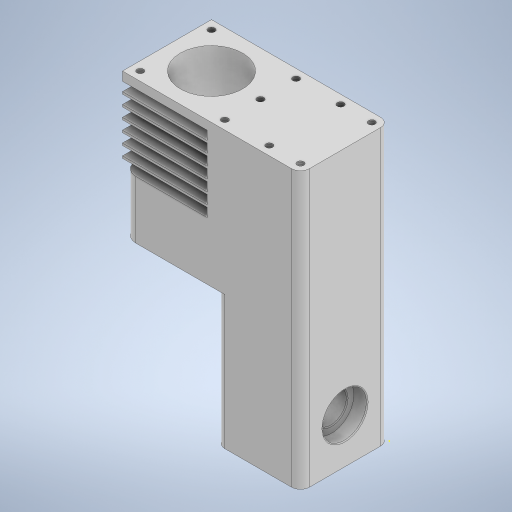
# Autodesk Inventor part: Hộp Piston
Saved by Autodesk Inventor 2023 (Build 270158000, 158)
## iProperties
Created: 2023-10-06
Part Number: Hộp Piston
Material: Generic
Document SubType Name: Modeling
Designer: huy20
Density: 1 g/cm^3
Appearance: Default
Author: huy20
Autodesk Inventor part; units mm, degrees
ref_plane "YZ Plane" through (0, 0, 0) normal (1, 0, 0) x (0, 1, 0)
ref_plane "XZ Plane" through (0, 0, 0) normal (0, 1, 0) x (-1, 0, 0)
sketch "Sketch1" plane through (0, 0, 0) normal (0, 0, 1) x (1, 0, 0)
  line L0 (0, 0) -> (19, 0)
  line L1 (0, 30) -> (0, 0)
  line L2 (0, 30) -> (-21, 30)
  line L3 (-21, 30) -> (-21, 62)
  line L4 (-21, 62) -> (19, 62)
  line L5 (19, 62) -> (19, 0)
  dimension "d0" = 32
  dimension "d1" = 21
  dimension "d2" = 30
  dimension "d3" = 40
  constraints: 12 end point, 2 horizontal, 2 perpendicular, 1 parallel
  measures "d0" distance of L2.end L3.end
  measures "d1" distance between parallel lines of L3 L1
  measures "d2" distance of L1.start L0.start
  measures "d3" distance of L3.end L4.end
extrude "Extrusion1" add sketch "Sketch1" along normal blind 20
sketch "Sketch2" plane through (-21, 30, 0) normal (0, -1, 0) x (1, 0, 0)
  circle A0 centre (10, 10) radius 7
  line L0 (0, 0) -> (21, 0) projected
  line L1 (0, 0) -> (0, 20) projected
  dimension "d6" = 14
  dimension "d7" = 10
  dimension "d8" = 10
  constraints: 1 centre point
  measures "d6" diameter of A0
  measures "d7" distance from line of L0 A0.centre
  measures "d8" distance from line of L1 A0.centre
extrude "Extrusion2" cut sketch "Sketch2" against normal through all
ref_plane "Work Plane1" through (-21, 60, 0) normal (0, 1, 0) x (1, 0, 0)
sketch "Sketch3" plane through (-21, 60, 0) normal (0, 1, 0) x (1, 0, 0)
  line L0 (0, 0) -> (0, -20) projected
  line L1 (21, 0) -> (0, 0)
  line L2 (0, 0) -> (0, -20)
  line L3 (0, -20) -> (19, -20)
  line L4 (2, -2) -> (20.5, -2)
  line L5 (18.5, -18) -> (2, -18)
  line L6 (2, -18) -> (2, -2)
  line L7 (20.5, -2) -> (21, -2)
  line L8 (18.5, -18) -> (19, -18)
  line L9 (19, -20) -> (19, -18)
  line L10 (21, -2) -> (21, 0)
  dimension "d12" = 2
  dimension "d13" = 2
  constraints: 20 end point, 6 perpendicular, 4 parallel, 1 horizontal, 1 other
  measures "d12" distance between parallel lines of L1 L4
  measures "d13" distance between parallel lines of L3 L5
extrude "Extrusion3" cut sketch "Sketch3" against normal blind 2
pattern_linear "Rectangular Pattern1" count 7 spacing 2.5 along (0, -1, 0) of "Extrusion3"
fillet "Fillet1" radius 3 16 edges at (-19, 59, 2) (-19, 56.5, 2) (-19, 54, 2) (-19, 51.5, 2) (-19, 49, 2) (-19, 46.5, 2) (-19, 44, 2) (-21, 36.5, 0) (-21, 36.5, 20) (-19, 44, 18) (-19, 46.5, 18) (-19, 49, 18) (-19, 51.5, 18) (-19, 54, 18) (-19, 56.5, 18) (-19, 59, 18)
fillet "Fillet2" radius 2 4 edges at (19, 31, 0) (19, 31, 20) (0, 15, 20) (0, 15, 0)
sketch "Sketch4" plane through (19, 0, 18) normal (1, 0, 0) x (0, 0, -1)
  line L0 (0, 0) -> (0, 62) construction
  line L1 (16, 0) -> (0, 0) construction
  line L2 (16, 62) -> (16, 0) construction
  line L3 (16, 62) -> (0, 62) construction
  circle A0 centre (8, 10) radius 3.5
  point P0 (18, 0)
  point P1 (8, 0)
  dimension "d21" = 7
  dimension "d22" = 10
  constraints: 1 centre point, 1 midpoint
  measures "d21" diameter of A0
  measures "d22" distance of point (8, 0) A0.centre
extrude "Extrusion4" cut sketch "Sketch4" against normal through all
sketch "Sketch5" plane through (-21, 62, 20) normal (0, 1, 0) x (1, 0, 0)
  circle A0 centre (10, 10) radius 7 projected
  arc A1 (38, 0) -> (40, 2) centre (38, 2) ccw projected
  line L0 (40, 18) -> (40, 2) projected
  arc A2 (40, 18) -> (38, 20) centre (38, 18) ccw projected
  line L1 (38, 20) -> (0, 20) projected
  line L2 (0, 20) -> (0, 0) projected
  line L3 (38, 0) -> (0, 0) projected
  line L4 (21, 18) -> (21, 2) projected
  point P0 (31, 18)
  point P1 (31, 2)
  point P2 (21, 10)
  point P3 (2, 18)
  point P4 (2, 2)
  dimension "d79" = 10
  dimension "d80" = 7
  dimension "d81" = 10
  dimension "d82" = 7
  dimension "d83" = 19
  dimension "d84" = 19
  dimension "d85" = 16
  dimension "d86" = 19
  dimension "d87" = 10
  dimension "d88" = 38
  constraints: 2 coincident
  measures "d79" distance of point (31, 18) L4.start
  measures "d80" distance of A2.centre point (31, 18)
  measures "d81" distance of point (31, 2) L4.end
  measures "d82" distance of A1.centre point (31, 2)
  measures "d83" distance of L4.end point (2, 2)
  measures "d84" distance of L4.start point (2, 18)
  measures "d85" distance of point (2, 2) point (2, 18)
  measures "d86" distance from line of point (21, 10) L0
  measures "d87" distance from line of point (21, 10) L1
  measures "d88" distance from line of point (2, 18) L0
hole "Hole1" at (0, 62, 2) at (-19, 62, 2) at (-19, 62, 18) at (0, 62, 18) at (10, 62, 18) at (17, 62, 18) at (17, 62, 2) at (10, 62, 2) at (0, 62, 10) direction (0, -1, 0) diameter 1.5 depth 3
sketch "Sketch6" plane through (2, 0, 0) normal (0, -1, 0) x (1, 0, 0)
  arc A0 (-2, 2) -> (0, 0) centre (0, 2) ccw projected
  line L0 (0, 0) -> (15, 0) projected
  arc A1 (15, 0) -> (17, 2) centre (15, 2) ccw projected
  line L1 (17, 2) -> (17, 18) projected
  arc A2 (17, 18) -> (15, 20) centre (15, 18) ccw projected
  line L2 (0, 20) -> (15, 20) projected
  arc A3 (0, 20) -> (-2, 18) centre (0, 18) ccw projected
  line L3 (-2, 2) -> (-2, 18) projected
  circle A4 centre (3, 10) radius 2
  circle A5 centre (11, 10) radius 2
  point P0 (-2, 0)
  dimension "d66" = 10
  dimension "d67" = 5
  dimension "d68" = 13
  dimension "d69" = 10
  dimension "d70" = 8
  dimension "d71" = 4
  dimension "d72" = 4
  constraints: 2 centre point
  measures "d66" distance from line of L2 A4.centre
  measures "d67" distance from line of L3 A4.centre
  measures "d68" distance from line of L3 A5.centre
  measures "d69" distance from line of L2 A5.centre
  measures "d70" distance of A4.centre A5.centre
  measures "d71" diameter of A4
  measures "d72" diameter of A5
extrude "Extrusion5" cut sketch "Sketch6" against normal blind 6 contours A4 | A5
thread "Thread11" size "M4x0.7" class "6H" standard "ANSI Metric M Profile" length 21
thread "Thread12" size "M4x0.7" class "6H" standard "ANSI Metric M Profile" length 21
thread "Thread13" size "M1.6x0.35" class "6H" standard "ANSI Metric M Profile" length 21
thread "Thread14" size "M1.6x0.35" class "6H" standard "ANSI Metric M Profile" length 21
thread "Thread15" size "M1.6x0.35" class "6H" standard "ANSI Metric M Profile" length 21
thread "Thread16" size "M1.6x0.35" class "6H" standard "ANSI Metric M Profile" length 21
thread "Thread17" size "M1.6x0.35" class "6H" standard "ANSI Metric M Profile" length 21
thread "Thread18" size "M1.6x0.35" class "6H" standard "ANSI Metric M Profile" length 21
thread "Thread19" size "M1.6x0.35" class "6H" standard "ANSI Metric M Profile" length 21
thread "Thread20" size "M1.6x0.35" class "6H" standard "ANSI Metric M Profile" length 21
thread "Thread21" size "M1.6x0.35" class "6H" standard "ANSI Metric M Profile" length 21
sketch "Sketch7" plane through (19, 0, 18) normal (1, 0, 0) x (0, 0, -1)
  point P0 (18, 0)
sketch "Sketch9" plane through (19, 0, 18) normal (1, 0, 0) x (0, 0, -1)
  circle A0 centre (8, 10) radius 3.5 projected
  circle A1 centre (8, 10) radius 3.5
  circle A2 centre (8, 10) radius 5
  point P0 (18, 0)
  dimension "d110" = 10
  constraints: 2 centre point, 2 coincident
  measures "d110" diameter of A2
extrude "Extrusion7" cut sketch "Sketch9" against normal blind 3
sketch "Sketch10" plane through (0, 0, 2) normal (-1, 0, 0) x (0, 0, 1)
  circle A0 centre (8, 10) radius 3.5 projected
  circle A1 centre (8, 10) radius 3.5
  circle A2 centre (8, 10) radius 5
  point P0 (-2, 0)
  dimension "d113" = 10
  constraints: 2 centre point, 2 coincident
  measures "d113" diameter of A2
extrude "Extrusion8" cut sketch "Sketch10" against normal blind 3
fillet "Fillet4" radius 0.2 3 edges at (19, 10, 15) (0, 10, 5) (16, 10, 13.5)
body "Solid1"
